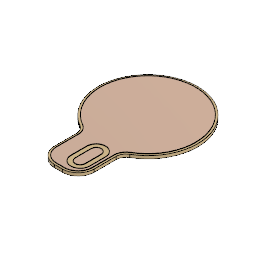
Z probe PCB (Autodesk Fusion 360 design; units mm, degrees)
Autodesk Fusion 360 part; units mm, degrees
sketch "Sketch1" plane through (0, 0, 0) normal (0, 0, 1) x (1, 0, 0)
  circle A0 centre (0, 0) radius 25
  line L0 (10, -45) -> (-10, -45)
  line L1 (-10, -45) -> (-10, 45)
  line L2 (-10, 45) -> (10, 45)
  line L3 (10, 45) -> (10, -45)
  line L4 (10, -45) -> (-10, 45) construction
  line L5 (-10, -45) -> (10, 45) construction
  dimension "d1" = 50
  dimension "d2" = 90
  dimension "d3" = 20
  constraint coincident A0.centre origin
  constraint perpendicular L0 L1
  constraint parallel L0 L2
  constraint parallel L1 L3
  constraint horizontal L0
  constraint coincident L4 A0.centre
  constraint coincident L5 A0.centre
  measures "d1" diameter of A0
  measures "d2" distance of L0.end L1.end
  measures "d3" distance of L1.end L2.end
extrude "Extrude1" add sketch "Sketch1" against normal blind 1.5 contours A0 L3 | A0 L1 L3 | A0 L0 L1 L3 | A0 L1
fillet "Fillet1" radius 8 2 edges at (-10, -45, -0.75) (10, -45, -0.75)
fillet "Fillet2" radius 5 2 edges at (-10, -22.9129, -0.75) (10, -22.9129, -0.75)
sketch "Sketch2" plane through (0, 0, 0) normal (0, 0, 1) x (-1, 0, 0)
  line L0 (-10, 37) -> (-10, 25.9808)
  arc A0 (-12.5, 21.6506) -> (12.5, 21.6506) centre (0, 0) ccw
  line L1 (10, 25.9808) -> (10, 37)
  line L2 (2, 45) -> (-2, 45)
  line L3 (-10, 33) -> (-3, 33)
  line L4 (-0.5, 28.9564) -> (-0.5, 37.0436)
  arc A1 (-0.5, 37.0436) -> (-5.5, 37.0436) centre (-3, 37.0436) ccw
  line L5 (-5.5, 37.0436) -> (-5.5, 28.9564)
  arc A2 (-5.5, 28.9564) -> (-0.5, 28.9564) centre (-3, 28.9564) ccw
  line L6 (-3, 28.9564) -> (-3, 37.0436) construction
  line L7 (1.7, 28.9564) -> (1.7, 37.0436)
  arc A3 (1.7, 37.0436) -> (-7.7, 37.0436) centre (-3, 37.0436) ccw
  line L8 (-7.7, 37.0436) -> (-7.7, 28.9564)
  arc A4 (-7.7, 28.9564) -> (1.7, 28.9564) centre (-3, 28.9564) ccw
  arc A5 (-2, 45) -> (-10, 37) centre (-2, 37) ccw
  arc A6 (-12.5, 21.6506) -> (-10, 25.9808) centre (-15, 25.9808) ccw
  arc A7 (10, 25.9808) -> (12.5, 21.6506) centre (15, 25.9808) ccw
  arc A8 (10, 37) -> (2, 45) centre (2, 37) ccw
  line L9 (-9, 37) -> (-9, 25.9808)
  arc A9 (-12, 20.7846) -> (-9, 25.9808) centre (-15, 25.9808) ccw
  arc A10 (-12, 20.7846) -> (12, 20.7846) centre (0, 0) ccw
  arc A11 (9, 25.9808) -> (12, 20.7846) centre (15, 25.9808) ccw
  line L10 (9, 25.9808) -> (9, 37)
  arc A12 (9, 37) -> (2, 44) centre (2, 37) ccw
  line L11 (2, 44) -> (-2, 44)
  arc A13 (-2, 44) -> (-9, 37) centre (-2, 37) ccw
  point P0 (-3, 33)
  dimension "d6" = 7
  dimension "d7" = 5
  dimension "d8" = 2.2
  dimension "d14" = 1
  constraint perpendicular L0 L3
  constraint tangent L4 A1
  constraint tangent A1 L5
  constraint parallel L4 L5
  constraint tangent L5 A2
  constraint tangent L4 A2
  constraint perpendicular L3 L6
  constraint coincident P0 L3.end
  constraint midpoint L6 P0
  constraint coincident L0 L3.start
  measures "d6" distance of L3.start P0
  measures "d7" diameter of A1
extrude "Extrude2" add sketch "Sketch2" along normal blind 0.2 contours L4 A1 L5 A2 | L9 A9 A10 A11 L10 A12 L11 A13
